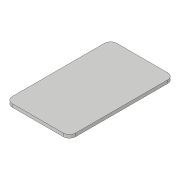
# Autodesk Inventor part: Activity 1 Custom Outline
Saved by Autodesk Inventor 2019 (Build 230136000, 136)
## iProperties
Created: 2020-04-18
Part Number: Activity 1 Custom Outline
Material: Generic
Document SubType Name: Modeling
Designer: Parthiv
Density: 1 g/cm^3
Appearance: Default
Author: Parthiv
Autodesk Inventor part; units mm, degrees
ref_plane "YZ Plane" through (0, 0, 0) normal (1, 0, 0) x (0, 1, 0)
ref_plane "XZ Plane" through (0, 0, 0) normal (0, 1, 0) x (-1, 0, 0)
ref_plane "XY Plane" through (0, 0, 0) normal (0, 0, 1) x (1, 0, 0)
sketch "Sketch1" plane through (0, 0, 0) normal (0, 1, 0) x (-1, 0, 0)
  line L0 (0, 0) -> (50.8, 0)
  line L1 (50.8, 0) -> (50.8, -83.82)
  line L2 (50.8, -83.82) -> (0, -83.82)
  line L3 (0, -83.82) -> (0, 0)
  dimension "d0" = 50.8
  dimension "d1" = 83.82
  constraints: 8 end point, 2 parallel, 1 horizontal, 1 perpendicular
  measures "d0" distance of L1.end L2.end
  measures "d1" distance of L0.end L1.end
extrude "Extrusion1" add sketch "Sketch1" along normal blind 2.54
fillet "Fillet1" radius 5 4 edges at (-50.8, 1.27, 0) (0, 1.27, 0) (0, 1.27, -83.82) (-50.8, 1.27, -83.82)
body "Solid1"
